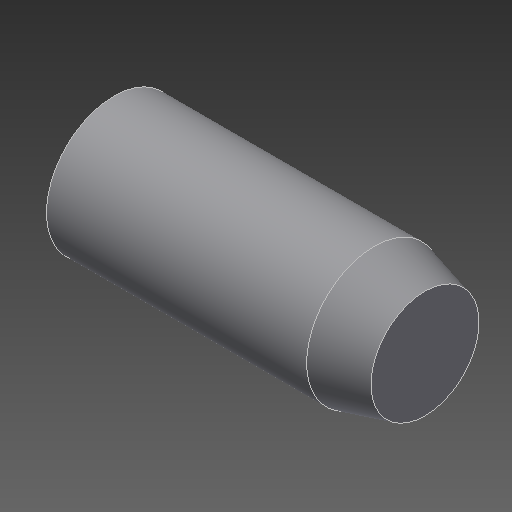
# Autodesk Inventor part: MS4-10
Saved by Autodesk Inventor 2021.1 (Build 251245010, 245A)
## iProperties
Created: 2010-03-11
Part Number: MS4-10
Catalog Web Link: www.cadenas.de
Document SubType Name: Modeling
Density: 1 g/cm^3
Material: MISUMI
Appearance: 既定
Category: PARTsolutions
NB: MS4-10
NN: MS, MSC
NT: Dowel Pins - Straight
NBSYN: $PN.
LINA: MS4-10
PN: MS4-10
TYPE: MS
MAT: 52100 Bearing Steel
HARD: 58HRC~
D: 4
D0: 1,1.5,2,2.5,3,4,5,6,8,10,12,13
L: 10
LL1: 1.5
L0: 8,10,15,20,25,30,35,40,45,50
MATALG: '','SUJ2(52100 Bearing Steel)(1.3505_100Cr6)','C','SUS440C(440C Stainless Steel)(1.4125_X105CrMo17)'
KT: DUMMY
PSOL_IDENT_0: {\\10.0.0.149\dplatte\cadenas\23d-libs\misumi\metric\28_keys_magnets\ms.prj},149 {VTYP=3D},{NB=MS4-1
PSOL_IDENT_1: 0},{LINA=MS4-10},{NN=MS, MSC},{DATE=26.05.2009 11:32:49},{GEOMDATE=21.04.2009},{VERSION=},{LINEID=10
PSOL_IDENT_2: },{LINESUBID=-1},{WBVAR=D,L}  {NB=MS4-10},{LINA=MS4-10},{KT=DUMMY},{PN=MS4-10},{TYPE=MS},{MAT=52100
PSOL_IDENT_3: Bearing Steel},{HARD=58HRC~},{D=4},{D0=1,1.5,2,2.5,3,4,5,6,8,10,12,13},{L=10},{LL1=1.5},{L0=8,10,15,
PSOL_IDENT_4: 20,25,30,35,40,45,50},{MATALG='','SUJ2(52100 Bearing Steel)(1.3505_100Cr6)','C','SUS440C(440C Stainl
PSOL_IDENT_5: ess Steel)(1.4125_X105CrMo17)'}
Title: ノックピン
Comments: Dowel Pins - Straight
Autodesk Inventor part; units mm, degrees
ref_plane "YZ Plane" through (0, 0, 0) normal (1, 0, 0) x (0, 1, 0)
ref_plane "XZ Plane" through (0, 0, 0) normal (0, 1, 0) x (-1, 0, 0)
ref_plane "XY Plane" through (0, 0, 0) normal (0, 0, 1) x (1, 0, 0)
sketch "Sketch_1" plane through (0, 0, 0) normal (0, 0, 1) x (1, 0, 0)
  line L0 (5, 0) -> (-5, 0)
  arc A0 (-4.2, 2) -> (-5, 0) centre (-1.0233, -0.4307) ccw
  line L1 (-4.2, 2) -> (3.5, 2)
  line L2 (3.5, 2) -> (5, 1.5981)
  line L3 (5, 1.5981) -> (5, 0)
  line L4 (5, 0) -> (-5, 0)
  constraints: 10 end point, 2 point on circle, 1 centre point
revolve "Revolution1" add sketch "Sketch_1" angle 360 about axis through (5, 0, 0) along (1, 0, 0)
